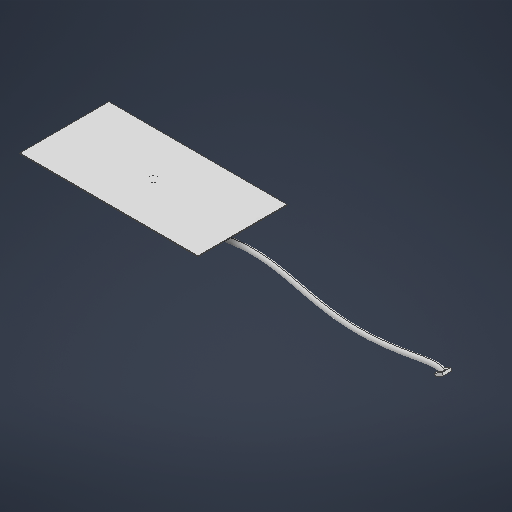
# Autodesk Inventor part: Antena
Saved by Autodesk Inventor 2027 (Build 310192000, 192)
## iProperties
Created: 2026-07-03
Part Number: Antena
Material: Genérico
Document SubType Name: Modeling
Designer: marcu
Density: 1 g/cm^3
Appearance: Padrão
Author: marcu
Autodesk Inventor part; units mm, degrees
ref_plane "YZ Plane" through (0, 0, 0) normal (1, 0, 0) x (0, 1, 0)
ref_plane "XZ Plane" through (0, 0, 0) normal (0, 1, 0) x (-1, 0, 0)
sketch "Esboço1" plane through (0, 0, 0) normal (0, 1, 0) x (1, 0, 0)
  line L0 (-20, 10) -> (20, 10)
  line L1 (20, 10) -> (20, -10)
  line L2 (20, -10) -> (-20, -10)
  line L3 (-20, -10) -> (-20, 10)
  line L4 (-20, 10) -> (20, -10) construction
  line L5 (20, 10) -> (-20, -10) construction
  point P0 (0, 0)
  dimension "d0" = 40
  dimension "d1" = 20
  constraints: 12 end point, 2 midpoint, 2 parallel, 1 horizontal, 1 perpendicular
  measures "d0" distance of L1.end L2.end
  measures "d1" distance of L0.end L1.end
extrude "Extrusão1" add sketch "Esboço1" along normal mid plane 0.15
sketch "Esboço2" plane through (0, 0, 0) normal (0, 0, 1) x (1, 0, 0)
  spline S0 degree 4 poles (0, 0) (8.3541, -9.8111) (24.1875, 8.376) (36.7418, -15.686) (63.5484, -2.469) (65, -5) knots 0 0 0 0 0 0.522164 1 1 1 1 1
  point P0 (13, -4)
  point P1 (25, -3)
  point P2 (40, -6)
  point P3 (59, -5)
  dimension "d7" = 65
  dimension "d8" = 6
  dimension "d9" = 19
  dimension "d10" = 15
  dimension "d11" = 12
  dimension "d12" = 4
  dimension "d13" = 3
  dimension "d14" = 6
  dimension "d15" = 5
  dimension "d17" = 5
  constraints: 6 other
  measures "d7" horizontal distance of point (65, -5) point (0, 0)
  measures "d8" distance of point (65, -5) point (59, -5)
  measures "d9" horizontal distance of point (59, -5) point (40, -6)
  measures "d10" horizontal distance of point (40, -6) point (25, -3)
  measures "d11" horizontal distance of point (25, -3) point (13, -4)
  measures "d12" vertical distance of point (13, -4) point (0, 0)
  measures "d13" vertical distance of point (25, -3) point (0, 0)
  measures "d14" vertical distance of point (0, 0) point (40, -6)
  measures "d15" vertical distance of point (59, -5) point (0, 0)
  measures "d17" vertical distance of point (65, -5) point (0, 0)
ref_plane "Plano de trabalho1" through (0, 0, 0) normal (0.6483, -0.7614, 0) x (0.7614, 0.6483, 0)
sketch "Esboço3" plane through (0, 0, 0) normal (0.6483, -0.7614, 0) x (0.7614, 0.6483, 0)
  circle A0 centre (0, 0) radius 0.565
  dimension "d4" = 1.13
  constraints: 1 centre point, 1 coincident
  measures "d4" diameter of A0
sweep "Varredura1" add profiles "Esboço3" path "Esboço2"
sketch "Esboço4" plane through (0, -0.075, 0) normal (0, -1, 0) x (1, 0, 0)
  circle A0 centre (0, 0) radius 1
  dimension "d18" = 2
  constraints: 1 centre point, 1 coincident
  measures "d18" diameter of A0
extrude "Extrusão2" add sketch "Esboço4" along normal mid plane 1
sketch "Esboço5" plane through (0, 0.075, 0) normal (0, 1, 0) x (1, 0, 0)
  line L0 (-1.25, 1.25) -> (1.25, 1.25)
  line L1 (1.25, 1.25) -> (1.25, -1.25)
  line L2 (1.25, -1.25) -> (-1.25, -1.25)
  line L3 (-1.25, -1.25) -> (-1.25, 1.25)
  arc A0 (0.8636, 0.5042) -> (0.8636, -0.5042) centre (0, 0) ccw projected
  line L4 (-1.25, 1.25) -> (1.25, -1.25) construction
  line L5 (1.25, 1.25) -> (-1.25, -1.25) construction
  dimension "d21" = 2.5
  dimension "d22" = 2.5
  constraints: 12 end point, 2 midpoint, 2 parallel, 1 horizontal, 1 perpendicular
  measures "d21" distance of L1.end L2.end
  measures "d22" distance of L0.end L1.end
extrude "Extrusão3" cut sketch "Esboço5" along normal blind 0.6
sketch "Esboço6" plane through (65, -5, 0) normal (0.4975, -0.8675, 0) x (0.8675, 0.4975, 0)
  line L0 (-1, -1) -> (1, -1)
  line L1 (1, -1) -> (1, 1)
  line L2 (1, 1) -> (-1, 1)
  line L3 (-1, 1) -> (-1, -1)
  circle A0 centre (0, 0) radius 0.565 projected
  line L4 (-1, -1) -> (1, 1) construction
  line L5 (1, -1) -> (-1, 1) construction
  point P0 (-53.8975, 0)
  point P1 (0.565, 0)
  dimension "d25" = 2
  dimension "d26" = 2
  constraints: 12 end point, 2 midpoint, 2 parallel, 1 horizontal, 1 horizontal alignment, 1 perpendicular
  measures "d25" distance of L1.end L2.end
  measures "d26" distance of L1.end L0.end
extrude "Extrusão4" add sketch "Esboço6" along normal mid plane 0.6 contours L3 L2 L1 L0 | A0
